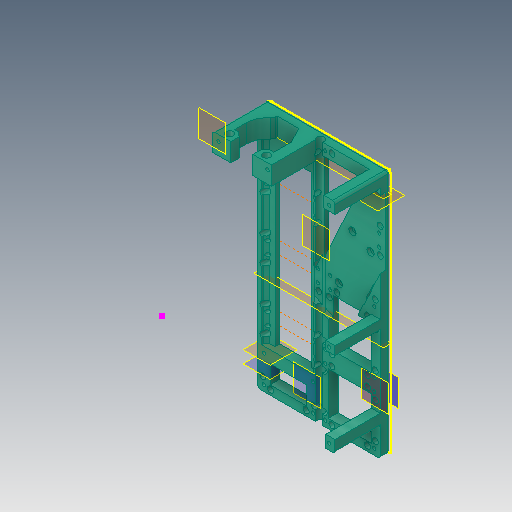
# Autodesk Inventor part: 30_CUBE_openSIM_base_v4
Saved by Autodesk Inventor 2019.4 (Build 234330000, 330)
## iProperties
Created: 2019-07-01
Part Number: 30_CUBE_openSIM_base_v4
Material: Generic
Document SubType Name: Modeling
Designer: diederichbenedict
Density: 1 g/cm^3
Appearance: IPHT_Türkis
Author: diederichbenedict
Autodesk Inventor part; units mm, degrees
ref_plane "YZ Plane" through (0, 0, 0) normal (1, 0, 0) x (0, 1, 0)
ref_plane "Work Plane15" through (181.6, 41.8, 16) normal (0, 0, -1) x (-1, 0, 0)
sketch "Sketch1" plane through (181.6, 41.8, 16) normal (0, 0, -1) x (-1, 0, 0)
  circle A0 centre (0.9, -0.9) radius 1.45 construction
  line L0 (4, -1.5) -> (1.5, -4) construction
  line L1 (4, -1.5) -> (4, 4) construction
  line L2 (4, 4) -> (-2, 4) construction
  arc A1 (-2, 4) -> (-4, 2) centre (-2, 2) ccw construction
  line L3 (-4, 2) -> (-4, -4) construction
  line L4 (-4, -4) -> (1.5, -4) construction
  arc A2 (45.8, 2) -> (43.8, 4) centre (43.8, 2) ccw construction
  line L5 (43.8, 4) -> (37.8, 4) construction
  line L6 (37.8, 4) -> (37.8, -1.5) construction
  line L7 (40.3, -4) -> (45.8, -4) construction
  line L8 (45.8, -4) -> (45.8, 2) construction
  circle A3 centre (40.9, -0.9) radius 1.45 construction
  line L9 (37.8, -40.3) -> (40.3, -37.8) construction
  line L10 (37.8, -40.3) -> (37.8, -45.8) construction
  line L11 (37.8, -45.8) -> (43.8, -45.8) construction
  arc A4 (43.8, -45.8) -> (45.8, -43.8) centre (43.8, -43.8) ccw construction
  line L12 (45.8, -43.8) -> (45.8, -37.8) construction
  line L13 (45.8, -37.8) -> (40.3, -37.8) construction
  circle A5 centre (40.9, -40.9) radius 1.45 construction
  circle A6 centre (0.9, -40.9) radius 1.45 construction
  line L14 (1.5, -37.8) -> (4, -40.3) construction
  line L15 (1.5, -37.8) -> (-4, -37.8) construction
  line L16 (-4, -37.8) -> (-4, -43.8) construction
  arc A7 (-4, -43.8) -> (-2, -45.8) centre (-2, -43.8) ccw construction
  line L17 (-2, -45.8) -> (4, -45.8) construction
  line L18 (4, -45.8) -> (4, -40.3) construction
  line L19 (40.3, -4) -> (37.8, -1.5) construction
  line L20 (-2, 154) -> (93.8, 154)
  line L21 (95.8, 152) -> (95.8, -43.8)
  line L22 (93.8, -45.8) -> (-2, -45.8)
  line L23 (-4, -43.8) -> (-4, 152)
  line L24 (90.3, -37.8) -> (90.3, 146)
  line L25 (87.8, 148.5) -> (4, 148.5)
  line L26 (1.5, 146) -> (1.5, -37.8)
  line L27 (4, -40.3) -> (87.8, -40.3)
  line L28 (87.8, -40.3) -> (90.3, -37.8)
  line L29 (4, -40.3) -> (1.5, -37.8)
  line L30 (4, 148.5) -> (1.5, 146)
  line L31 (90.3, 146) -> (87.8, 148.5)
  arc A8 (95.8, 152) -> (93.8, 154) centre (93.8, 152) ccw
  arc A9 (-2, 154) -> (-4, 152) centre (-2, 152) ccw
  circle A10 centre (1, -1) radius 1.4
  circle A11 centre (40.9, -0.9) radius 1.4
  circle A12 centre (90.9, -40.9) radius 1.4
  circle A13 centre (0.9, -40.9) radius 1.4
  circle A14 centre (45.9, 104.1) radius 44.4 construction
  line L32 (45.8, -37.8) -> (87.8, -37.8)
  line L33 (87.8, -37.8) -> (87.8, 146)
  line L34 (45.9, 148.5) -> (45.9, -40.3)
  line L35 (87.8, 146) -> (45.9, 146)
  line L36 (77.4, 111.7) -> (64.2, 111.7) construction
  line L37 (64.2, 96.7) -> (77.4, 96.7) construction
  line L38 (77.4, 61.7) -> (64.2, 61.7) construction
  line L39 (64.2, 46.7) -> (77.4, 46.7) construction
  line L40 (45.9, 111.7) -> (87.8, 111.7)
  line L41 (87.8, 111.7) -> (87.8, 96.7)
  line L42 (87.8, 96.7) -> (45.9, 96.7)
  line L43 (45.9, 96.7) -> (45.9, 111.7)
  line L44 (45.9, 61.7) -> (87.8, 61.7)
  line L45 (87.8, 61.7) -> (87.8, 46.7)
  line L46 (87.8, 46.7) -> (45.9, 46.7)
  line L47 (45.9, 46.7) -> (45.9, 61.7)
  line L48 (95.8, -43.8) -> (95.8, -45.8)
  line L49 (95.8, -45.8) -> (93.8, -45.8)
  line L50 (-4, -43.8) -> (-4, -45.8)
  line L51 (-4, -45.8) -> (-2, -45.8)
  point P0 (95.8, 154)
  point P1 (90.3, -40.3)
  point P2 (90.3, 148.5)
  point P3 (1.5, 148.5)
  point P4 (1.5, -40.3)
  point P5 (40.8, 149)
  point P6 (45.8, -40.8)
  point P7 (45.9, -37.8)
  point P8 (63.2, 61.7)
  dimension "d34" = 99.8
  dimension "d35" = 199.8
  dimension "d36" = 5.5
  dimension "d37" = 2.5
  dimension "d38" = 2.5
  dimension "d39" = 2.5
  dimension "d40" = 2.5
  dimension "d41" = 2.5
  dimension "d42" = 2.5
  dimension "d43" = 2.5
  dimension "d44" = 2.5
  dimension "d45" = 2
  dimension "d46" = 4.9
  dimension "d47" = 4.9
  dimension "d48" = 4.9
  dimension "d49" = 4.9
  dimension "d50" = 5
  dimension "d51" = 5
  dimension "d52" = 0.5
  dimension "d53" = 5
  dimension "d54" = 5
  dimension "d55" = 2.8
  dimension "d56" = 2.8
  dimension "d57" = 2.8
  dimension "d58" = 2.8
  constraints: 56 end point, 22 point on line, 9 coincident, 9 parallel, 7 perpendicular, 6 centre point, 5 horizontal, 5 tangent, 4 point on circle, 3 midpoint, 2 vertical, 1 equal radius, 1 vertical alignment, 6 other
  measures "d34" distance of point (95.8, -45.8) L50.end
  measures "d35" distance of point (95.8, 154) point (95.8, -45.8)
  measures "d36" distance between parallel lines of L21 L24
  measures "d37" distance of L27.end point (90.3, -40.3)
  measures "d38" distance of L24.start point (90.3, -40.3)
  measures "d39" distance of L27.start point (1.5, -40.3)
  measures "d40" distance of L26.end point (1.5, -40.3)
  measures "d41" distance of L25.end point (1.5, 148.5)
  measures "d42" distance of L26.start point (1.5, 148.5)
  measures "d43" distance of L24.end point (90.3, 148.5)
  measures "d44" distance of L25.start point (90.3, 148.5)
  measures "d45" radius of A8
  measures "d46" distance from line of point (0.9, -40.9) L23
  measures "d47" distance from line of L22 point (0.9, -40.9)
  measures "d48" distance from line of L21 point (90.9, -40.9)
  measures "d49" distance from line of L22 point (90.9, -40.9)
  measures "d50" distance from line of L8 point (40.8, 149)
  measures "d51" distance from line of L20 point (40.8, 149)
  measures "d52" distance from line of point (1, -1) L26
  measures "d53" distance from line of L3 point (1, -1)
  measures "d54" distance from line of L2 point (1, -1)
  measures "d55" diameter of A10
  measures "d56" diameter of A11
  measures "d57" diameter of A12
  measures "d58" diameter of A13
extrude "Extrusion1" add sketch "Sketch1" along normal blind 8 contours L20 A8 L21 L48 L49 L22 L51 L50 L23 A9 | L28 L27 L34 L32 L33 L35 L25 L31 L24 | L27 L29 L26 A10 L30 L25 L34 | L34 L44 L33 L46 | L40 L33 L42 L34 | L26 A10 | A11 picked at (1.6831, -0.6911)
ref_plane "Work Plane16" through (181.6, 41.8, 8) normal (0, 0, -1) x (-1, 0, 0)
sketch "Sketch4" plane through (181.6, 41.8, 8) normal (0, 0, -1) x (-1, 0, 0)
  line L0 (-4, -45.8) -> (95.8, -45.8) construction
  line L1 (4, -37.8) -> (4, 146) construction
  circle A0 centre (1, -40.8) radius 1.4 construction
  line L2 (1, -1) -> (41, -1) construction
  line L3 (41, -1) -> (41, -41) construction
  line L4 (41, -41) -> (1, -41) construction
  line L5 (1, -41) -> (1, -1) construction
  line L6 (-4, 154) -> (95.8, 154)
  line L7 (95.8, 154) -> (95.8, -45.8)
  line L8 (95.8, -45.8) -> (-4, -45.8)
  line L9 (-4, -45.8) -> (-4, 154)
  line L10 (95.8, 152) -> (95.8, -45.8) projected
  line L11 (95.8, 53.1) -> (-4, 53.1)
  line L12 (-4, -45.8) -> (-4, 152) projected
  line L13 (95.8, 53.1) -> (195.6, 53.1) construction
  circle A1 centre (0.9, 59.1) radius 1.4
  circle A2 centre (0.9, 99.1) radius 1.4
  circle A3 centre (40.9, 59.1) radius 1.4
  circle A4 centre (40.9, 99.1) radius 1.4
  circle A5 centre (0.9, 149.1) radius 1.4
  circle A6 centre (40.9, 149.1) radius 1.4
  circle A7 centre (40.9, 109.1) radius 1.4
  circle A8 centre (0.9, 109.1) radius 1.4
  circle A9 centre (50.9, 99.1) radius 1.4
  circle A10 centre (90.9, 99.1) radius 1.4
  circle A11 centre (90.9, 59.1) radius 1.4
  circle A12 centre (50.9, 59.1) radius 1.4
  circle A13 centre (50.9, 149.1) radius 1.4
  circle A14 centre (90.9, 149.1) radius 1.4
  circle A15 centre (90.9, 109.1) radius 1.4
  circle A16 centre (50.9, 109.1) radius 1.4
  circle A17 centre (0.9, 49.1) radius 1.4
  circle A18 centre (40.9, 9.1) radius 1.4
  circle A19 centre (0.9, 9.1) radius 1.4
  circle A20 centre (40.9, 49.1) radius 1.4
  circle A21 centre (0.9, -0.9) radius 1.4
  circle A22 centre (0.9, -40.9) radius 1.4
  line L14 (41, -1) -> (41, -41) construction
  circle A23 centre (40.9, -40.9) radius 1.4
  circle A24 centre (40.9, -0.9) radius 1.4
  line L15 (-4, -95.8) -> (-4, 104)
  circle A25 centre (50.9, 49.1) radius 1.4
  circle A26 centre (50.9, 9.1) radius 1.4
  line L16 (91, 49) -> (91, 9) construction
  circle A27 centre (90.9, 9.1) radius 1.4
  circle A28 centre (90.9, 49.1) radius 1.4
  line L17 (46, -45.8) -> (46, 154)
  circle A29 centre (50.9, -0.9) radius 1.4
  circle A30 centre (50.9, -40.9) radius 1.4
  line L18 (91, -1) -> (91, -41) construction
  circle A31 centre (90.9, -40.9) radius 1.4
  circle A32 centre (90.9, -0.9) radius 1.4
  line L19 (46, -95.8) -> (46, 104)
  point P0 (1, -40.8)
  point P1 (1, -1)
  point P2 (-2, -45.8)
  point P3 (1, -40.8)
  point P4 (41, 9)
  point P5 (41, 49)
  point P6 (-4, 102)
  point P7 (46, 152)
  point P8 (46, 102)
  dimension "d479" = 99.8
  dimension "d482" = 2.8
  dimension "d483" = 6
  dimension "d484" = 4.9
  dimension "d487" = 40
  dimension "d490" = 40
  dimension "d495" = 50
  dimension "d498" = 50
  dimension "d503" = 50
  dimension "d510" = 50
  dimension "d513" = 50
  constraints: 33 centre point, 32 end point, 6 horizontal, 4 parallel, 4 vertical, 3 perpendicular, 2 coincident, 1 collinear, 1 midpoint, 81 other
  measures "d479" distance of L11.start L11.end
  measures "d482" diameter of A1
  measures "d483" distance from line of L11 A1.centre
  measures "d484" distance from line of L12 A1.centre
  measures "d487" distance of A1.centre A2.centre
  measures "d490" distance of A1.centre A3.centre
  measures "d495" distance of A2.centre A5.centre
  measures "d498" distance of A2.centre A9.centre
  measures "d503" distance of A2.centre A17.centre
  measures "d510" distance of A17.centre A21.centre
  measures "d513" distance of A17.centre A25.centre
sketch "Sketch23" plane through (181.6, 41.8, 16) normal (0, 0, 1) x (1, 0, 0)
  line L0 (-87.8, 111.7) -> (-45.9, 111.7) projected
  line L1 (-87.8, 111.7) -> (-87.8, 146) projected
  line L2 (-87.8, 146) -> (-45.9, 146) projected
  line L3 (-45.9, 146) -> (-45.9, 111.7) projected
  line L4 (-45.9, 96.7) -> (-45.9, 61.7) projected
  line L5 (-87.8, 61.7) -> (-45.9, 61.7) projected
  line L6 (-87.8, 61.7) -> (-87.8, 96.7) projected
  line L7 (-45.9, 96.7) -> (-87.8, 96.7) projected
  line L8 (-45.9, -37.8) -> (-87.8, -37.8) projected
  line L9 (-87.8, -37.8) -> (-87.8, 46.7) projected
  line L10 (-45.9, 46.7) -> (-87.8, 46.7) projected
  line L11 (-45.9, 46.7) -> (-45.9, -37.8) projected
  line L12 (-95.8, 152) -> (-95.8, -45.8) projected
  line L13 (-95.8, -45.8) -> (4, -45.8) projected
  line L14 (4, -45.8) -> (4, 152) projected
  arc A0 (4, 152) -> (2, 154) centre (2, 152) ccw projected
  line L15 (2, 154) -> (-93.8, 154) projected
  arc A1 (-93.8, 154) -> (-95.8, 152) centre (-93.8, 152) ccw projected
  point P0 (-181.6, -41.8)
extrude "Extrusion15" add sketch "Sketch23" against normal up to surface (8 mm away) contours L1 L2 L3 L0 | L4 L5 L6 L7 | L8 L9 L10 L11
sketch "Sketch26" plane through (181.6, 41.8, 16) normal (0, 0, -1) x (-1, 0, 0)
  arc A0 (7.0096, 100.7998) -> (7.6791, 99.3501) centre (6.3003, 99.5928) ccw construction
  line L0 (19.4325, 78.671) -> (-0.7895, 122.4569) construction
  circle A1 centre (21.0984, 106.427) radius 1.4 construction
  line L1 (10.811, 105.155) -> (33.6759, 57.326) construction
  circle A2 centre (33.6759, 57.326) radius 2.1706
  circle A3 centre (3.6505, 101.3448) radius 1.4
  arc A4 (19.4922, 109.1893) -> (19.7163, 108.7194) centre (18.3626, 108.3621) ccw
  line L2 (18.3626, 108.3621) -> (3.6505, 101.3448)
  line L3 (11.0066, 104.8535) -> (33.6998, 57.2762)
  line L4 (18.3626, 108.3621) -> (3.6505, 101.3448) construction
  line L5 (3.6505, 101.3448) -> (0.9579, 106.9899) construction
  line L6 (0.9579, 106.9899) -> (15.67, 114.0073) construction
  line L7 (15.67, 114.0073) -> (18.3626, 108.3621) construction
  line L8 (18.3626, 108.3621) -> (3.6505, 101.3448) construction
  line L9 (3.6505, 101.3448) -> (7.9556, 92.319) construction
  line L10 (7.9556, 92.319) -> (22.6677, 99.3363) construction
  line L11 (22.6677, 99.3363) -> (18.3626, 108.3621) construction
  point P0 (181.6, -41.8)
  point P1 (3.5305, 101.5964)
  point P2 (18.2427, 108.6137)
  point P3 (18.2427, 108.6137)
  dimension "d266" = 90
  dimension "d267" = 8.15
  dimension "d268" = 10
  constraints: 22 end point, 5 equal length, 3 centre point, 2 coincident, 2 perpendicular, 2 point on circle, 1 midpoint, 1 point on line, 8 other
  measures "d266" angle of L2 L3
  measures "d267" distance from line of L2.start L3
  measures "d268" distance of L9.end L2.end
ref_plane "Work Plane6" through (183.6, 180.8, 16) normal (0, 1, 0) x (-1, 0, 0)
ref_plane "Work Plane7" through (183.6, 75.8, 16) normal (0, 1, 0) x (-1, 0, 0)
sketch "Sketch29" plane through (181.6, 41.8, 8) normal (0, 0, -1) x (-1, 0, 0)
  point P0 (181.6, -41.8)
ref_plane "Work Plane17" through (181.6, 41.8, 16) normal (0, 0, 1) x (1, 0, 0)
sketch "Sketch30" plane through (181.6, 41.8, 16) normal (0, 0, 1) x (1, 0, 0)
  arc A0 (4, 152) -> (2, 154) centre (2, 152) ccw projected
  line L0 (2, 154) -> (-93.8, 154) projected
  arc A1 (-93.8, 154) -> (-95.8, 152) centre (-93.8, 152) ccw projected
  line L1 (-95.8, -45.8) -> (4, -45.8) projected
  line L2 (6.5, -43.3) -> (-43.3, -43.3) construction
  line L3 (-43.3, -43.3) -> (-43.3, 6.5) construction
  line L4 (-43.3, 6.5) -> (6.5, 6.5) construction
  line L5 (6.5, 6.5) -> (6.5, -43.3) construction
  line L6 (-93.3, -43.3) -> (-43.5, -43.3) construction
  line L7 (-43.5, -43.3) -> (-43.5, 6.5) construction
  line L8 (-43.5, 6.5) -> (-93.3, 6.5) construction
  line L9 (-93.3, 6.5) -> (-93.3, -43.3) construction
  line L10 (-56.9142, 124) -> (-85.811, 124) construction
  line L11 (-81.9373, 124) -> (-81.9373, 139) construction
  line L12 (-56.9142, 124) -> (-81.9373, 124) construction
  line L13 (-56.9142, 139) -> (-56.9142, 124) construction
  line L14 (-56.9142, 139) -> (-81.9373, 139) construction
  circle A2 centre (-69.55, -19.75) radius 26.25 construction
  line L15 (-38.4, -38.5) -> (-3.4, -38.5) construction
  line L16 (-3.4, -38.5) -> (-3.4, -3.5) construction
  line L17 (-3.4, -3.5) -> (-38.4, -3.5) construction
  line L18 (-38.4, -3.5) -> (-38.4, -38.5) construction
  line L19 (-38.4, -38.5) -> (-3.4, -3.5) construction
  line L20 (-3.4, -38.5) -> (-38.4, -3.5) construction
  line L21 (-38.4, -3.5) -> (-3.4, -3.5)
  line L22 (-3.4, -3.5) -> (-3.4, -38.5)
  line L23 (-3.4, -38.5) -> (-38.4, -38.5)
  line L24 (-38.4, -38.5) -> (-38.4, -3.5)
  line L25 (-38.4, -3.5) -> (-3.4, -38.5) construction
  line L26 (-3.4, -3.5) -> (-38.4, -38.5) construction
  line L27 (6.5, 6.5) -> (-43.3, 6.5)
  line L28 (-43.3, 6.5) -> (-43.3, 56.3)
  line L29 (-43.3, 56.3) -> (6.5, 56.3)
  line L30 (6.5, 56.3) -> (6.5, 6.5) construction
  line L31 (-3.4, 46.3229) -> (-38.4, 46.3229)
  line L32 (-38.4, 46.3229) -> (-38.4, 11.3229)
  line L33 (-38.4, 11.3229) -> (-3.4, 11.3229)
  line L34 (-3.4, 11.3229) -> (-3.4, 46.3229)
  line L35 (-3.4, 46.3229) -> (-38.4, 11.3229) construction
  line L36 (-38.4, 46.3229) -> (-3.4, 11.3229) construction
  line L37 (-55.8, -38.5) -> (-85.8, -38.5)
  line L38 (-85.8, -38.5) -> (-85.8, 6.5)
  line L39 (-85.8, 6.5) -> (-55.8, 6.5)
  line L40 (-55.8, 6.5) -> (-55.8, -38.5)
  line L41 (-7.9405, 76.5555) -> (-34.9278, 89.4278) projected
  line L42 (-10.9392, 144.6427) -> (-45.9, 144.6427)
  line L43 (-45.9, 144.6427) -> (-45.9, 71.4872)
  line L44 (-55.8, 124) -> (-85.8, 124)
  line L45 (-85.8, 124) -> (-85.8, 34)
  line L46 (-55.8, 34) -> (-55.8, 124)
  line L47 (-55.8, 6.5) -> (-85.8, 6.5)
  line L48 (-85.8, 6.5) -> (-85.8, 19)
  line L49 (-55.8, 19) -> (-55.8, 6.5)
  line L50 (-10.9392, 144.6427) -> (-45.9, 68.723)
  line L51 (-45.9, 68.723) -> (-45.9, 71.4872)
  line L52 (4, -45.8) -> (4, 152) projected
  line L53 (-95.8, 152) -> (-95.8, -45.8) projected
  line L54 (-1, 9) -> (-41.0771, 49) construction
  line L55 (-85.8, 19) -> (-85.8, 34)
  line L56 (-55.8, 34) -> (-55.8, 19)
  point P0 (-181.6, -41.8)
  point P1 (-90.5546, 19)
  point P2 (-90.5546, 34)
  point P3 (-45.8, 34)
  point P4 (-45.8, 19)
  point P5 (-20.9, -21)
  point P6 (-20.9, -21)
  dimension "d191" = 49.8
  dimension "d192" = 49.8
  dimension "d193" = 49.8
  dimension "d194" = 49.8
  dimension "d196" = 35
  dimension "d197" = 35
  dimension "d198" = 49.8
  dimension "d199" = 35
  dimension "d200" = 35
  dimension "d205" = 45
  constraints: 94 end point, 17 parallel, 10 horizontal, 10 perpendicular, 5 midpoint, 2 point on line, 2 tangent, 2 vertical, 1 centre point, 1 collinear
  measures "d191" distance of L3.end L4.end
  measures "d192" distance of L2.end L3.end
  measures "d193" distance of L8.end L7.end
  measures "d194" distance of L7.end L6.end
  measures "d196" distance of L17.end L16.end
  measures "d197" distance of L16.end L15.end
  measures "d198" distance of L27.end L28.end
  measures "d199" distance of L33.end L32.end
  measures "d200" distance of L32.end L31.end
  measures "d205" distance of L37.end L38.end
extrude "Extrusion19" cut sketch "Sketch30" against normal blind 15 contours L21 L22 L23 L24 | L34 L33 L32 L31 | L37 L38 L39 L40 | L39 L48 L55 L45 L44 L46 L56 L49 | L50 L51 L43 L42
ref_plane "Work Plane28" through (183.6, 180.8, 16) normal (0, 1, 0) x (-1, 0, 0)
sketch "Sketch31" plane through (183.6, 180.8, 16) normal (0, 1, 0) x (-1, 0, 0)
  circle A0 centre (47.8, -1.2) radius 3.1
  line L0 (97.8, -1.7) -> (97.8, -4.5) projected
  line L1 (97.8, 0) -> (-2, 0) projected
  point P0 (183.6, -16)
  point P1 (95.8, 0)
  point P2 (0, 0)
  point P3 (-2, 0)
  dimension "d207" = 6.2
  dimension "d208" = 50
  dimension "d209" = 1.2
  constraints: 1 centre point, 1 other
  measures "d207" diameter of A0
  measures "d208" distance from line of A0.centre L0
extrude "Extrusion20" cut sketch "Sketch31" along normal through all both and the other way through all
ref_plane "Work Plane18" through (181.6, 41.8, 8) normal (0, 0, -1) x (-1, 0, 0)
sketch "Sketch36" plane through (181.6, 41.8, 8) normal (0, 0, -1) x (-1, 0, 0)
  line L0 (90.8, -40.8) -> (51, -40.8) construction
  line L1 (51, -40.8) -> (51, -1) construction
  line L2 (51, -1) -> (90.8, -1) construction
  line L3 (90.8, -1) -> (90.8, -40.8) construction
  line L4 (91, 9) -> (51, 9) construction
  line L5 (51, 9) -> (51, 49) construction
  line L6 (51, 49) -> (91, 49) construction
  line L7 (91, 49) -> (91, 9) construction
  line L8 (91, 59) -> (51, 59) construction
  line L9 (51, 59) -> (51, 99) construction
  line L10 (51, 99) -> (91, 99) construction
  line L11 (91, 99) -> (91, 59) construction
  line L12 (-4, -45.8) -> (95.8, -45.8) projected
  line L13 (93.8, 154) -> (-2, 154) projected
  arc A0 (-2, 154) -> (-4, 152) centre (-2, 152) ccw projected
  line L14 (-4, 152) -> (-4, -45.8) projected
  line L15 (95.8, -45.8) -> (95.8, 152) projected
  arc A1 (95.8, 152) -> (93.8, 154) centre (93.8, 152) ccw projected
  point P0 (181.6, -41.8)
  point P1 (49.923, -2.077)
  point P2 (49.923, 9)
  constraints: 24 end point, 6 parallel, 3 horizontal, 3 perpendicular, 2 coincident
hole "Hole13" at (180.7, 190.9, 8) at (140.7, 190.9, 8) at (130.7, 190.9, 8) at (90.7, 190.9, 8) at (180.7, 150.9, 8) at (180.7, 140.9, 8) at (130.7, 140.9, 8) at (130.7, 150.9, 8) at (90.7, 150.9, 8) at (90.7, 140.9, 8) at (140.7, 100.9, 8) at (130.7, 100.9, 8) at (90.7, 100.9, 8) at (90.7, 90.9, 8) at (130.7, 90.9, 8) at (140.7, 90.9, 8) at (180.7, 90.9, 8) at (180.7, 100.9, 8) at (140.7, 50.9, 8) at (90.7, 40.9, 8) at (90.7, 50.9, 8) at (130.7, 50.9, 8) at (130.7, 40.9, 8) at (180.7, 0.9, 8) at (140.7, 0.9, 8) at (130.7, 0.9, 8) at (90.7, 0.9, 8) at (180.7, 40.9, 8) at (180.7, 50.9, 8) at (140.7, 40.9, 8) direction (0, 0, 1) diameter 2.8 depth 12 tip angle 118 counterbore diameter 6 counterbore depth 2.5
hole "Hole11" at (158.9323, 141.1363, 16) at (173.6444, 134.119, 16) at (147.9241, 99.126, 16) direction (0, 0, -1) diameter 2.7 end through all counterbore diameter 6 counterbore depth 6.5
sketch "Sketch41" plane through (181.6, 41.8, 16) normal (0, 0, 1) x (1, 0, 0)
  line L0 (21.4433, 131.7452) -> (-28.6669, 26.687)
  line L1 (-28.6669, 26.687) -> (-60.8287, 42.0274)
  line L2 (-60.8287, 42.0274) -> (-10.7185, 147.0856)
  line L3 (-10.7185, 147.0856) -> (21.4433, 131.7452)
  constraints: 8 end point, 2 parallel, 1 perpendicular
extrude "Extrusion24" cut sketch "Sketch41" against normal blind 4
ref_plane "Work Plane21" through (181.6, 41.8, 16) normal (0, 0, 1) x (1, 0, 0)
sketch "Sketch43" plane through (181.6, 41.8, 16) normal (0, 0, 1) x (1, 0, 0)
  line L0 (-38.4, 31.3294) -> (-42.9417, 33.4957) projected
  line L1 (4, -45.8) -> (4, 95.1746) projected
  line L2 (4, 95.1746) -> (-19.3011, 46.3229) projected
  line L3 (-9.0689, 56.7246) -> (-3.3295, 68.7575)
  line L4 (-3.3295, 68.7575) -> (-5.8525, 69.9609)
  line L5 (-5.8525, 69.9609) -> (-11.5918, 57.928)
  line L6 (-11.5918, 57.928) -> (-9.0689, 56.7246)
  line L7 (4, 95.1746) -> (-19.3011, 46.3229) projected
  line L8 (-95.8, 152) -> (-95.8, -45.8) projected
  line L9 (-11.8837, 144.6427) -> (-10.7185, 147.0856) projected
  line L10 (-10.7185, 147.0856) -> (4, 140.0653) projected
  line L11 (4, 140.0653) -> (4, 152) projected
  arc A0 (4, 152) -> (2, 154) centre (2, 152) ccw projected
  line L12 (2, 154) -> (-42.9417, 154) projected
  line L13 (-42.9417, -45.8) -> (4, -45.8) projected
  arc A1 (-93.8, 154) -> (-95.8, 152) centre (-93.8, 152) ccw projected
  line L14 (-55.8, 52.5702) -> (-48.6583, 67.5431) projected
  line L15 (-48.6583, 67.5431) -> (-48.6583, 154) projected
  line L16 (-48.6583, 154) -> (-93.8, 154) projected
  line L17 (-48.6583, -45.8) -> (-48.6583, 36.2224) projected
  line L18 (-95.8, -45.8) -> (-48.6583, -45.8) projected
  line L19 (-42.9417, 154) -> (-42.9417, 144.6427) projected
  line L20 (-42.9417, 33.4957) -> (-42.9417, -45.8) projected
  line L21 (-48.6583, 36.2224) -> (-55.8, 39.6288) projected
  line L22 (-55.8, 39.6288) -> (-55.8, -38.5) projected
  line L23 (-55.8, -38.5) -> (-85.8, -38.5) projected
  line L24 (-85.8, -38.5) -> (-85.8, 124) projected
  line L25 (-85.8, 124) -> (-55.8, 124) projected
  line L26 (-55.8, 124) -> (-55.8, 52.5702) projected
  line L27 (-42.9417, 144.6427) -> (-11.8837, 144.6427) projected
  line L28 (-19.3011, 46.3229) -> (-3.4, 46.3229) projected
  line L29 (-3.4, 46.3229) -> (-3.4, 11.3229) projected
  line L30 (-3.4, 11.3229) -> (-38.4, 11.3229) projected
  line L31 (-38.4, 11.3229) -> (-38.4, 31.3294) projected
  circle A2 centre (-40.9, -0.9) radius 1.4 projected
  point P0 (-181.6, -41.8)
  constraints: 8 end point, 3 parallel, 1 perpendicular
extrude "Extrusion26" cut sketch "Sketch43" against normal through all contours L6 L5 L4 L3
ref_plane "Work Plane20" through (181.6, 41.8, 8) normal (0, 0, -1) x (-1, 0, 0)
ref_plane "Work Plane23" through (132.9417, 125.8, 16) normal (0, 0, 1) x (1, 0, 0)
ref_plane "Work Plane27" through (85.8, 195.8, 52.921) normal (0, 0, 1) x (1, 0, 0)
ref_plane "Work Plane11" through (95.3202, 23.1, 15.4189) normal (0, 1, 0) x (0, 0, 1)
ref_plane "Work Plane12" through (74.6511, 18.1, -2.2213) normal (0, -1, 0) x (1, 0, 0)
sketch "Sketch53" plane through (87.8, 195.8, 8) normal (0, 1, 0) x (1, 0, 0)
  line L0 (-2, -8) -> (-2, -44.921) projected
  line L1 (-2, -44.921) -> (13, -44.921) projected
  line L2 (13, -44.921) -> (13, -34.921) projected
  line L3 (13, -34.921) -> (8, -34.921) projected
  line L4 (6, -32.921) -> (6, -24.8366) projected
  line L5 (6, -24.8366) -> (13.8224, -9.1093) projected
  line L6 (32.1358, -9.1093) -> (38, -20.8998) projected
  line L7 (38, -20.8998) -> (38, -32.921) projected
  line L8 (36, -34.921) -> (31, -34.921) projected
  line L9 (31, -34.921) -> (31, -44.921) projected
  line L10 (31, -44.921) -> (46, -44.921) projected
  arc A0 (45.1417, -8) -> (46, -9.1685) centre (48, -6.8) ccw projected
  line L11 (46, -44.921) -> (46, -9.1685) projected
  line L12 (6, -32.921) -> (6, -34.921)
  line L13 (6, -34.921) -> (8, -34.921)
  line L14 (36, -34.921) -> (38, -34.921)
  line L15 (38, -34.921) -> (38, -32.921)
  line L16 (13.8224, -9.1093) -> (14.3742, -8)
  line L17 (32.1358, -9.1093) -> (31.584, -8)
  arc A1 (46.6696, -4) -> (45.1417, -8) centre (48, -6.8) ccw projected
  line L18 (31.584, -8) -> (45.1417, -8)
  line L19 (-2, -8) -> (-2, 0) projected
  line L20 (14.3742, -8) -> (-2, -8)
  circle A2 centre (7, -39.921) radius 3.1
  circle A3 centre (37, -39.921) radius 3.1
  point P0 (-87.8, 8)
  point P1 (0, 0)
  dimension "d417" = 6.2
  dimension "d418" = 6.2
  constraints: 16 end point, 2 centre point, 2 horizontal, 2 perpendicular, 1 point on line, 1 vertical
  measures "d417" diameter of A2
  measures "d418" diameter of A3
extrude "Extrusion37" add sketch "Sketch53" against normal blind 15
fillet "Fillet8" radius 2 1 edges at (85.8, 195.8, 34.4605)
ref_plane "Work Plane30" through (95.8, 18.1, 16) normal (0, -1, 0) x (1, 0, 0)
sketch "Sketch55" plane through (87.8, 195.8, 8) normal (0, 1, 0) x (1, 0, 0)
  line L0 (3.657, -45.987) -> (40.343, -45.987)
  line L1 (40.343, -45.987) -> (43.066, -43.264)
  line L2 (43.066, -43.264) -> (43.066, -6.578)
  line L3 (43.066, -6.578) -> (40.343, -3.855)
  line L4 (40.343, -3.855) -> (3.657, -3.855)
  line L5 (3.657, -3.855) -> (0.934, -6.578)
  line L6 (0.934, -6.578) -> (0.934, -43.264)
  line L7 (0.934, -43.264) -> (3.657, -45.987)
  point P0 (-87.8, 8)
  constraints: 16 end point
ref_plane "Work Plane34" through (125.8, 18.1, 16) normal (0, 0, -1) x (-1, 0, 0)
sketch "Sketch57" plane through (125.8, 18.1, 16) normal (0, 0, -1) x (-1, 0, 0)
  line L0 (0, 0) -> (30, 0) projected
  line L1 (0, 10) -> (-2.343, 10) projected
  line L2 (30, 0) -> (0, 0)
  line L3 (0, 0) -> (0, 10)
  line L4 (0, 10) -> (30, 10)
  line L5 (30, 10) -> (30, 0)
  point P0 (125.8, -18.1)
  constraints: 8 end point, 2 parallel, 1 horizontal, 1 perpendicular
extrude "Extrusion40" add sketch "Sketch57" along normal blind 8
sketch "Sketch64" plane through (181.6, 41.8, 16) normal (0, 0, 1) x (1, 0, 0)
  line L0 (4, -45.8) -> (4, 95.1746) projected
  line L1 (-3.4, -38.5) -> (-3.4, -3.5) projected
  line L2 (4, -23.7) -> (-3.4, -23.7)
  line L3 (-3.4, -23.7) -> (-3.4, -13.7)
  line L4 (-3.4, -13.7) -> (4, -13.7)
  line L5 (4, -13.7) -> (4, -23.7)
  line L6 (4, 154) -> (-5, 154)
  line L7 (-5, 154) -> (-5, 145)
  line L8 (-5, 145) -> (4, 145)
  line L9 (4, 145) -> (4, 154)
  line L10 (4, 152) -> (4, -45.8) projected
  line L11 (4, 52.5) -> (-3.4, 52.5)
  line L12 (-3.4, 52.5) -> (-3.4, 45.5)
  line L13 (-3.4, 45.5) -> (4, 45.5)
  line L14 (4, 45.5) -> (4, 52.5)
  point P0 (-181.6, -41.8)
  dimension "d398" = 10
  dimension "d404" = 9
  dimension "d405" = 9
  dimension "d419" = 7.4
  dimension "d420" = 7
  constraints: 24 end point, 6 parallel, 3 horizontal, 3 perpendicular, 3 point on line
  measures "d398" distance of L2.end L3.end
  measures "d404" distance of L8.end L7.end
  measures "d405" distance of L7.end L6.end
  measures "d419" distance of L13.end L12.end
  measures "d420" distance of L12.end L11.end
extrude "Extrusion42" add sketch "Sketch64" along normal blind 36.921
fillet "Fillet9" radius 2 1 edges at (185.6, 195.8, 34.4605)
sketch "Sketch50" plane through (85.8, 195.8, 52.921) normal (0, 0, 1) x (1, 0, 0)
  circle A0 centre (4.9, -4.9) radius 1.4
  circle A1 centre (44.9, -4.9) radius 1.4
  line L0 (2, 0) -> (15, 0) projected
  line L1 (0, -2) -> (0, -15) projected
  line L2 (33, 0) -> (48, 0) projected
  circle A2 centre (94.9, -4.9) radius 1.4
  line L3 (99.8, 0) -> (90.8, 0) projected
  line L4 (99.8, -9) -> (99.8, 0) projected
  circle A3 centre (94.9, -104.9) radius 1.4 projected
  circle A4 centre (94.9, -172.7) radius 1.4
  line L5 (99.8, -167.7) -> (92.4, -167.7) projected
  line L6 (99.8, -177.7) -> (99.8, -167.7) projected
  circle A5 centre (4.9, -172.7) radius 1.4
  circle A6 centre (44.9, -172.7) radius 1.4
  line L7 (0, -177.7) -> (0, -167.7) projected
  line L8 (0, -167.7) -> (48, -167.7) projected
  circle A7 centre (44.9, -194.9) radius 1.4 projected
  point P0 (-85.8, -195.8)
  point P1 (97.8, 0)
  point P2 (99.8, -2)
  dimension "d357" = 2.8
  dimension "d358" = 2.8
  dimension "d543" = 4.9
  dimension "d544" = 4.9
  dimension "d545" = 4.9
  dimension "d546" = 2.8
  dimension "d547" = 4.9
  dimension "d548" = 4.9
  dimension "d549" = 40
  dimension "d550" = 2.8
  dimension "d551" = 5
  dimension "d552" = 4.9
  dimension "d553" = 2.8
  dimension "d555" = 5
  dimension "d556" = 2.8
  dimension "d557" = 5
  dimension "d558" = 0
  dimension "d561" = 4.9
  constraints: 6 centre point
  measures "d357" diameter of A0
  measures "d358" diameter of A1
  measures "d543" distance from line of L0 A0.centre
  measures "d544" distance from line of L1 A0.centre
  measures "d545" distance from line of L2 A1.centre
  measures "d546" diameter of A2
  measures "d547" distance from line of L3 A2.centre
  measures "d548" distance from line of L4 A2.centre
  measures "d549" distance of A1.centre A0.centre
  measures "d550" diameter of A4
  measures "d551" distance from line of A4.centre L5
  measures "d552" distance from line of L6 A4.centre
  measures "d553" diameter of A5
  measures "d555" distance from line of L8 A5.centre
  measures "d556" diameter of A6
  measures "d557" distance from line of L8 A6.centre
  measures "d558" horizontal distance of A6.centre A7.centre
  measures "d561" distance from line of L7 A5.centre
extrude "Extrusion33" cut sketch "Sketch50" against normal through all contours A0 | A1 | A2 | A3 | A4 | A5 | A6
fillet "Fillet10" radius 2 4 edges at (185.6, 18.1, 34.4605) (185.6, -4, 12) (85.8, -4, 12) (135.7, -4, 8)
fillet "Fillet11" radius 2 7 edges at (185.0142, 195.2142, 8) (185.6, 95.9, 8) (185.0142, -3.4142, 8.5858) (86.3858, 195.2142, 8) (85.8, 95.9, 8) (86.3858, -3.4142, 8.5858) (135.7, 195.8, 8)
sketch "Sketch67" plane through (181.6, 41.8, 8) normal (0, 0, -1) x (-1, 0, 0)
  arc A0 (90.8, -43.8) -> (93.8, -40.8) centre (90.8, -40.8) ccw projected
  circle A1 centre (85.4, -41.7) radius 2.45
  circle A2 centre (91.7, -35.4) radius 2.45
  line L0 (91.7, -35.4) -> (101.7, -35.4) construction
  line L1 (91.7, -35.4) -> (91.7, -20.9)
  line L2 (92.866, -13.7) -> (90.143, -13.7) projected
  line L3 (91.7, -20.9) -> (70.9, -20.9)
  line L4 (70.9, -20.9) -> (70.9, -30.9)
  circle A3 centre (85.4, -0.1) radius 2.45
  circle A4 centre (91.7, -6.4) radius 2.45
  line L5 (-2, -45.8) -> (93.8, -45.8) projected
  line L6 (95.8, -43.8) -> (95.8, 152) projected
  circle A5 centre (56.4, -41.7) radius 2.45
  circle A6 centre (50.1, -35.4) radius 2.45
  circle A7 centre (50.1, -6.4) radius 2.45
  circle A8 centre (56.4, -0.1) radius 2.45
  circle A9 centre (56.4, 49.9) radius 2.45
  circle A10 centre (50.1, 43.6) radius 2.45
  circle A11 centre (91.7, 43.6) radius 2.45
  circle A12 centre (85.4, 49.9) radius 2.45
  circle A13 centre (56.4, 8.3) radius 2.45
  circle A14 centre (50.1, 14.6) radius 2.45
  circle A15 centre (85.4, 8.3) radius 2.45
  circle A16 centre (91.7, 14.6) radius 2.45
  line L7 (91.7, 14.6) -> (91.7, 29.1)
  circle A17 centre (56.4, 99.9) radius 2.45
  circle A18 centre (50.1, 93.6) radius 2.45
  circle A19 centre (91.7, 93.6) radius 2.45
  circle A20 centre (85.4, 99.9) radius 2.45
  circle A21 centre (56.4, 58.3) radius 2.45
  circle A22 centre (50.1, 64.6) radius 2.45
  circle A23 centre (85.4, 58.3) radius 2.45
  circle A24 centre (91.7, 64.6) radius 2.45
  line L8 (91.7, 64.6) -> (91.7, 79.1)
  circle A25 centre (56.4, 149.9) radius 2.45
  circle A26 centre (50.1, 143.6) radius 2.45
  circle A27 centre (91.7, 143.6) radius 2.45
  circle A28 centre (85.4, 149.9) radius 2.45
  circle A29 centre (56.4, 108.3) radius 2.45
  circle A30 centre (50.1, 114.6) radius 2.45
  circle A31 centre (85.4, 108.3) radius 2.45
  circle A32 centre (91.7, 114.6) radius 2.45
  line L9 (91.7, 114.6) -> (91.7, 129.1)
  circle A33 centre (6.4, -0.1) radius 2.45
  circle A34 centre (0.1, -6.4) radius 2.45
  circle A35 centre (41.7, -6.4) radius 2.45
  circle A36 centre (35.4, -0.1) radius 2.45
  circle A37 centre (6.4, -41.7) radius 2.45
  circle A38 centre (0.1, -35.4) radius 2.45
  circle A39 centre (35.4, -41.7) radius 2.45
  circle A40 centre (41.7, -35.4) radius 2.45
  line L10 (41.7, -35.4) -> (41.7, -20.9)
  circle A41 centre (6.4, 49.9) radius 2.45
  circle A42 centre (0.1, 43.6) radius 2.45
  circle A43 centre (41.7, 43.6) radius 2.45
  circle A44 centre (35.4, 49.9) radius 2.45
  circle A45 centre (6.4, 8.3) radius 2.45
  circle A46 centre (0.1, 14.6) radius 2.45
  circle A47 centre (35.4, 8.3) radius 2.45
  circle A48 centre (41.7, 14.6) radius 2.45
  line L11 (41.7, 14.6) -> (41.7, 29.1)
  circle A49 centre (6.4, 99.9) radius 2.45
  circle A50 centre (0.1, 93.6) radius 2.45
  circle A51 centre (41.7, 93.6) radius 2.45
  circle A52 centre (35.4, 99.9) radius 2.45
  circle A53 centre (6.4, 58.3) radius 2.45
  circle A54 centre (0.1, 64.6) radius 2.45
  circle A55 centre (35.4, 58.3) radius 2.45
  circle A56 centre (41.7, 64.6) radius 2.45
  line L12 (41.7, 64.6) -> (41.7, 79.1)
  circle A57 centre (6.4, 149.9) radius 2.45
  circle A58 centre (0.1, 143.6) radius 2.45
  circle A59 centre (41.7, 143.6) radius 2.45
  circle A60 centre (35.4, 149.9) radius 2.45
  circle A61 centre (6.4, 108.3) radius 2.45
  circle A62 centre (0.1, 114.6) radius 2.45
  circle A63 centre (35.4, 108.3) radius 2.45
  circle A64 centre (41.7, 114.6) radius 2.45
  line L13 (41.7, 114.6) -> (41.7, 129.1)
  point P0 (181.6, -41.8)
  dimension "d433" = 4.9
  dimension "d436" = 4.9
  dimension "d528" = 14.5
  dimension "d529" = 20.8
  dimension "d530" = 10
  dimension "d531" = 10.4
  dimension "d532" = 10.4
  dimension "d533" = 4.1
  dimension "d534" = 4.1
  dimension "d537" = 50
  dimension "d540" = 50
  constraints: 65 centre point, 22 end point, 6 symmetric about line, 2 horizontal, 2 perpendicular, 2 vertical, 1 collinear, 131 other
  measures "d433" diameter of A1
  measures "d436" diameter of A2
  measures "d528" distance of L0.start L1.end
  measures "d529" distance of L1.end L3.end
  measures "d530" distance of L3.end L4.end
  measures "d531" distance from line of L5 L0.start
  measures "d532" distance from line of L6 A1.centre
  measures "d533" distance from line of L6 L0.start
  measures "d534" distance from line of L5 A1.centre
  measures "d537" distance of A8.centre A9.centre
  measures "d540" distance of A8.centre A33.centre
extrude "Extrusion44" cut sketch "Sketch67" against normal blind 10 contours A1 | A2 | A4 | A5 | A6 | A7 | A10 | A11 | A14 | A16 | A18 | A19 | A24 | A25 | A26 | A27 | A28 | A30 | A32 | A33 | A34 | A35 | A36 | A37 | A38 | A39 | A40 | A41 | A42 | A43 | A44 | A45 | A46 | A47 | A48 | A50 | A54 | A57 | A58 | A60 | A62
sketch "Sketch74" plane through (181.6, 41.8, 52.921) normal (0, 0, 1) x (1, 0, 0)
  circle A0 centre (-0.9, 49.1) radius 1.4 projected
  circle A1 centre (-0.9, -18.7) radius 1.4 projected
  circle A2 centre (-0.9, 149.1) radius 1.4 projected
  point P0 (-181.6, -41.8)
extrude "Extrusion51" cut sketch "Sketch74" against normal through all
ref_plane "Work Plane35" through (95.8, 28.1, 16) normal (0, 1, 0) x (1, 0, 0)
sketch "Sketch76" plane through (95.8, 28.1, 16) normal (0, 1, 0) x (1, 0, 0)
  line L0 (7.3885, -20.2147) -> (18.1492, -9.454) projected
  line L1 (18.1492, -9.454) -> (22.9588, -14.2636) projected
  line L2 (22.9588, -14.2636) -> (12.1981, -25.0243) projected
  line L3 (12.1981, -25.0243) -> (7.3885, -20.2147) projected
  line L4 (18.1492, -9.454) -> (16.0279, -7.3327)
  line L5 (16.0279, -7.3327) -> (26.6345, -17.9393)
  line L6 (26.6345, -17.9393) -> (15.8738, -28.7)
  line L7 (15.8738, -28.7) -> (5.2672, -18.0934)
  line L8 (5.2672, -18.0934) -> (16.0279, -7.3327)
  point P0 (-95.8, 16)
  dimension "d266" = 90
  dimension "d565" = 3
  dimension "d566" = 15
  constraints: 10 end point, 2 parallel, 1 perpendicular, 1 point on line
  measures "d565" distance of L0.end L4.end
  measures "d566" distance of L4.end L5.end
extrude "Extrusion52" cut sketch "Sketch76" against normal blind 5 contours L7 L8 L4 L0 | L2 L5 L6 L7
sketch "Sketch77" plane through (102.1742, 195.8, 16) normal (0, 1, 0) x (1, 0, 0)
  circle A0 centre (7.6259, -16.921) radius 14.986 projected
  circle A1 centre (7.6259, -16.921) radius 15.986
  point P0 (-102.1742, 16)
  dimension "d571" = 1
  constraints: 1 centre point
  measures "d571" radial gap between concentric circles of A0 A1
extrude "Extrusion53" cut sketch "Sketch77" against normal blind 15 contours A0 | A1
extrude "Extrusion54" cut sketch "Sketch55" against normal up to surface (152.7 mm away) from surface at -15
sketch "Sketch78" plane through (181.6, 41.8, 16) normal (0, 0, 1) x (1, 0, 0)
  line L0 (9.6188, 100.4778) -> (-15.3507, 48.1278) projected
  line L1 (4, 85) -> (-14.448, 46.3229)
  line L2 (4, 52.5) -> (4, 95.1746) projected
  line L3 (4, 85) -> (4, 95.1746)
  line L4 (4, 95.1746) -> (-19.3011, 46.3229) projected
  line L5 (-19.3011, 46.3229) -> (-14.448, 46.3229)
  line L6 (-19.3011, 46.3229) -> (-3.4, 46.3229) projected
  point P0 (-181.6, -41.8)
  dimension "d574" = 1.5918
  constraints: 6 end point, 3 point on line, 1 parallel
  measures "d574" distance between parallel lines of L0 L1
extrude "Extrusion55" cut sketch "Sketch78" against normal up to surface (4 mm away) from surface at 0
equation "\"d38\" = d37"
equation "\"d39\" = d37"
equation "\"d40\" = d39"
equation "\"d41\" = d37"
equation "\"d42\" = d41"
equation "\"d43\" = d37"
equation "\"d44\" = d43"
body "Solid1"
